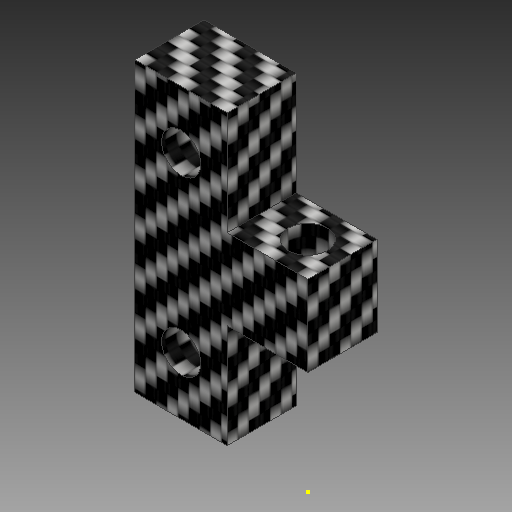
# Autodesk Inventor part: kamera ut
Saved by Autodesk Inventor 2018 (Build 220112000, 112)
## iProperties
Created: 2018-01-30
Part Number: kamera ut
Material: CFK
Document SubType Name: Modeling
Designer: Andreas
Density: 1.43 g/cm^3
Appearance: Kohlenstofffaser
Mass: 1.88974 g
Surface Area: 11.2647 cm^2
Volume: 1.3215 cm^3
Author: Andreas
Autodesk Inventor part; units mm, degrees
ref_plane "YZ Plane" through (0, 0, 0) normal (1, 0, 0) x (0, 1, 0)
ref_plane "XZ Plane" through (0, 0, 0) normal (0, 1, 0) x (-1, 0, 0)
ref_plane "XY Plane" through (0, 0, 0) normal (0, 0, 1) x (1, 0, 0)
sketch "Skizze1" plane through (0, 0, 0) normal (0, 1, 0) x (-1, 0, 0)
  line L0 (0, 0) -> (15, 0)
  line L1 (15, 0) -> (15, -25)
  line L2 (15, -25) -> (0, -25)
  line L3 (0, -25) -> (0, 0)
  dimension "d0" = 25
  dimension "d1" = 15
  constraints: 8 end point, 2 parallel, 1 horizontal, 1 perpendicular
  measures "d0" distance of L0.end L1.end
  measures "d1" distance of L1.end L2.end
extrude "Extrusion1" add sketch "Skizze1" along normal blind 6
sketch "Skizze3" plane through (0, 0, -25) normal (0, 0, -1) x (-1, 0, 0)
  point P0 (0, 0)
sketch "Skizze6" plane through (0, 6, 0) normal (0, 1, 0) x (1, 0, 0)
  circle A0 centre (-11, 5) radius 1.7
  line L0 (-15, 25) -> (-15, 0) projected
  line L1 (-15, 0) -> (0, 0) projected
  circle A1 centre (-11, 20) radius 1.7
  line L2 (0, 25) -> (-15, 25) projected
  point P0 (0, 30)
  dimension "d11" = 3.4
  dimension "d12" = 4
  dimension "d13" = 5
  dimension "d14" = 3.4
  dimension "d15" = 4
  dimension "d16" = 5
  constraints: 2 centre point, 1 other
  measures "d11" diameter of A0
  measures "d12" distance from line of L0 A0.centre
  measures "d13" distance from line of L1 A0.centre
  measures "d14" diameter of A1
  measures "d15" distance from line of L0 A1.centre
extrude "Extrusion4" cut sketch "Skizze6" against normal blind 30
sketch "Skizze7" plane through (0, 0, 0) normal (0, -1, 0) x (1, 0, 0)
  line L0 (0, -25) -> (-15, -25) projected
  line L1 (0, -25) -> (-7, -25)
  line L2 (-7, -25) -> (-7, -16)
  line L3 (-7, -16) -> (0, -16)
  line L4 (0, -16) -> (0, -25)
  line L5 (-15, 0) -> (0, 0) projected
  line L6 (0, 0) -> (-7, 0)
  line L7 (-7, 0) -> (-7, -9)
  line L8 (-7, -9) -> (0, -9)
  line L9 (0, -9) -> (0, 0)
  dimension "d19" = 7
  dimension "d20" = 9
  dimension "d21" = 7
  dimension "d22" = 9
  constraints: 16 end point, 4 parallel, 2 horizontal, 2 perpendicular
  measures "d19" distance of L2.end L3.end
  measures "d20" distance of L1.end L2.end
  measures "d21" distance of L7.end L8.end
  measures "d22" distance of L6.end L7.end
extrude "Extrusion5" cut sketch "Skizze7" against normal blind 30
sketch "Skizze8" plane through (-7, 0, -9) normal (0, 0, 1) x (1, 0, 0)
  circle A0 centre (4, 3) radius 1.7
  line L0 (7, 0) -> (0, 0) projected
  line L1 (7, 6) -> (7, 0) projected
  dimension "d25" = 3.4
  dimension "d26" = 3
  dimension "d27" = 3
  constraints: 1 centre point
  measures "d25" diameter of A0
  measures "d26" distance from line of L0 A0.centre
  measures "d27" distance from line of L1 A0.centre
extrude "Extrusion6" cut sketch "Skizze8" against normal blind 30
